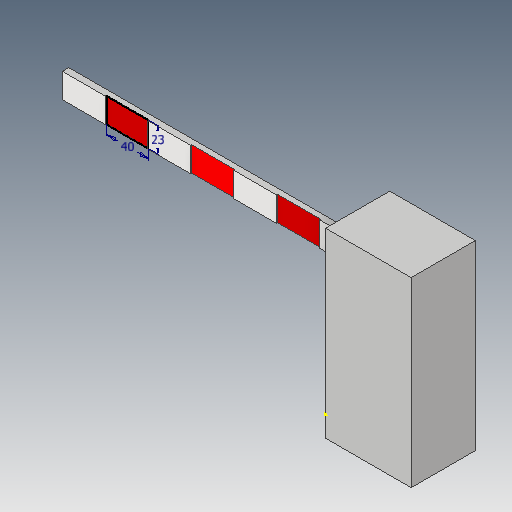
# Autodesk Inventor part: bar
Saved by Autodesk Inventor 2018 (Build 220112000, 112)
## iProperties
Created: 2017-08-24
Part Number: bar
Material: Generic
Document SubType Name: Modeling
Designer: Platform
Density: 1 g/cm^3
Appearance: Default
Author: Platform
Autodesk Inventor part; units mm, degrees
ref_plane "YZ Plane" through (0, 0, 0) normal (1, 0, 0) x (0, 1, 0)
ref_plane "XZ Plane" through (0, 0, 0) normal (0, 1, 0) x (-1, 0, 0)
ref_plane "XY Plane" through (0, 0, 0) normal (0, 0, 1) x (1, 0, 0)
sketch "Sketch1" plane through (0, 0, 0) normal (0, 0, 1) x (1, 0, 0)
  point P0 (0, 0)
sketch "Sketch2" plane through (0, 0, 0) normal (0, 0, 1) x (1, 0, 0)
  line L0 (-270, 130) -> (30, 130)
  line L1 (30, 130) -> (30, 107)
  line L2 (30, 107) -> (-270, 107)
  line L3 (-270, 107) -> (-270, 130)
  line L4 (0, 0) -> (80, 0)
  line L5 (80, 0) -> (80, 150)
  line L6 (80, 150) -> (0, 150)
  line L7 (0, 150) -> (0, 0)
  dimension "d0" = 300
  dimension "d1" = 23
  dimension "d2" = 80
  dimension "d3" = 150
  dimension "d4" = 30
  dimension "d5" = 20
  constraints: 16 end point, 4 parallel, 2 horizontal, 2 perpendicular
  measures "d0" distance of L1.end L2.end
  measures "d1" distance of L0.end L1.end
  measures "d2" distance of L6.end L5.end
  measures "d3" distance of L5.end L4.end
  measures "d4" distance between parallel lines of L1 L7
  measures "d5" distance between parallel lines of L6 L0
extrude "Extrusion1" add sketch "Sketch2" along normal mid plane 5 contours L0 L7 L2 L3 | L0 L1 L2 L7
sketch "Sketch3" plane through (0, 0, 2.5) normal (0, 0, 1) x (1, 0, 0)
  point P0 (0, 0)
sketch "Sketch4" plane through (0, 0, 2.5) normal (0, 0, 1) x (1, 0, 0)
  point P0 (0, 0)
sketch "Sketch5" plane through (0, 0, -2.5) normal (0, 0, -1) x (-1, 0, 0)
  line L0 (0, 0) -> (-80, 0)
  line L1 (-80, 0) -> (-80, 150)
  line L2 (-80, 150) -> (0, 150)
  line L3 (0, 150) -> (0, 0)
  dimension "d8" = 80
  dimension "d9" = 150
  constraints: 8 end point, 2 parallel, 1 horizontal, 1 perpendicular
  measures "d8" distance of L1.end L2.end
  measures "d9" distance of L0.end L1.end
extrude "Extrusion2" add sketch "Sketch5" along normal mid plane 60
sketch "Sketch6" plane through (0, 0, 2.5) normal (0, 0, 1) x (1, 0, 0)
  line L0 (-270, 107) -> (-270, 130) projected
  line L1 (-270, 130) -> (-230, 130)
  line L2 (-230, 130) -> (-230, 107)
  line L3 (-230, 107) -> (-270, 107)
  line L4 (-270, 107) -> (-270, 130)
  point P0 (0, 0)
  dimension "d12" = 40
  dimension "d13" = 23
  constraints: 8 end point, 2 parallel, 1 horizontal, 1 perpendicular
  measures "d12" distance of L2.end L3.end
  measures "d13" distance of L1.end L2.end
extrude "Extrusion3" add sketch "Sketch6" along normal blind 1
sketch "Sketch7" plane through (0, 0, 2.5) normal (0, 0, 1) x (1, 0, 0)
  line L0 (-230.0222, 129.8127) -> (-190.0222, 129.8127)
  line L1 (-190.0222, 129.8127) -> (-190.0222, 106.8127)
  line L2 (-190.0222, 106.8127) -> (-230.0222, 106.8127)
  line L3 (-230.0222, 106.8127) -> (-230.0222, 129.8127)
  point P0 (0, 0)
  dimension "d16" = 40
  dimension "d17" = 23
  constraints: 8 end point, 2 parallel, 1 horizontal, 1 perpendicular
  measures "d16" distance of L1.end L2.end
  measures "d17" distance of L0.end L1.end
sketch "Sketch8" plane through (0, 0, 2.5) normal (0, 0, 1) x (1, 0, 0)
  line L0 (-230, 107) -> (-230, 130) projected
  line L1 (-230, 130) -> (-190, 130)
  line L2 (-190, 130) -> (-190, 107)
  line L3 (-190, 107) -> (-230, 107)
  line L4 (-230, 107) -> (-230, 130)
  line L5 (-190, 130) -> (-150, 130)
  line L6 (-150, 130) -> (-150, 107)
  line L7 (-150, 107) -> (-190, 107)
  line L8 (-190, 107) -> (-190, 130)
  point P0 (0, 0)
  dimension "d18" = 40
  dimension "d19" = 23
  dimension "d20" = 40
  dimension "d21" = 23
  constraints: 16 end point, 4 parallel, 2 horizontal, 2 perpendicular
  measures "d18" distance of L2.end L3.end
  measures "d19" distance of L1.end L2.end
  measures "d20" distance of L6.end L7.end
  measures "d21" distance of L5.end L6.end
extrude "Extrusion4" add sketch "Sketch8" along normal blind 1 contours L2 L5 L6 L7
sketch "Sketch9" plane through (0, 0, 2.5) normal (0, 0, 1) x (1, 0, 0)
  line L0 (-150, 130) -> (-110, 130)
  line L1 (-110, 130) -> (-110, 107)
  line L2 (-110, 107) -> (-150, 107)
  line L3 (-150, 107) -> (-150, 130)
  line L4 (-110, 130) -> (-70, 130)
  line L5 (-70, 130) -> (-70, 107)
  line L6 (-70, 107) -> (-110, 107)
  line L7 (-110, 107) -> (-110, 130)
  point P0 (0, 0)
  dimension "d24" = 40
  dimension "d25" = 23
  dimension "d26" = 40
  dimension "d27" = 23
  constraints: 16 end point, 4 parallel, 2 horizontal, 2 perpendicular
  measures "d24" distance of L1.end L2.end
  measures "d25" distance of L0.end L1.end
  measures "d26" distance of L5.end L6.end
  measures "d27" distance of L4.end L5.end
extrude "Extrusion5" add sketch "Sketch9" along normal blind 1 contours L4 L5 L6 L1
sketch "Sketch10" plane through (0, 0, 2.5) normal (0, 0, 1) x (1, 0, 0)
  line L0 (-70, 130) -> (-70, 107) projected
  line L1 (-70, 130) -> (-30, 130)
  line L2 (-30, 130) -> (-30, 107)
  line L3 (-30, 107) -> (-70, 107)
  line L4 (-70, 107) -> (-70, 130)
  line L5 (0, 107) -> (0, 130) projected
  line L6 (-30, 130) -> (0, 130)
  line L7 (0, 130) -> (0, 107)
  line L8 (0, 107) -> (-30, 107)
  line L9 (-30, 107) -> (-30, 130)
  point P0 (0, 0)
  dimension "d30" = 40
  dimension "d31" = 23
  dimension "d32" = 30
  dimension "d33" = 23
  constraints: 16 end point, 4 parallel, 2 horizontal, 2 perpendicular
  measures "d30" distance of L2.end L3.end
  measures "d31" distance of L1.end L2.end
  measures "d32" distance of L5.start L8.end
  measures "d33" distance of L6.end L5.start
extrude "Extrusion6" add sketch "Sketch10" along normal blind 1 contours L6 L5 L8 L2
sketch "Sketch11" plane through (0, 0, 27.5) normal (0, 0, 1) x (1, 0, 0)
  point P0 (0, 0)
sketch "Sketch12" plane through (0, 0, 27.5) normal (0, 0, 1) x (1, 0, 0)
  line L0 (0, 0) -> (80, 0) projected
  line L1 (80, 0) -> (80, -20)
  line L2 (80, -20) -> (0, -20)
  line L3 (0, -20) -> (0, 0)
  dimension "d36" = 20
  constraints: 6 end point, 1 horizontal, 1 perpendicular, 1 vertical
  measures "d36" distance of L0.end L1.end
extrude "Extrusion7" add sketch "Sketch12" against normal blind 60
body "Solid1"
